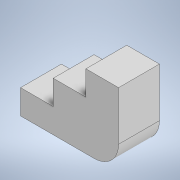
# Autodesk Inventor part: 1.4
Saved by Autodesk Inventor 2022 (Build 260153000, 153)
## iProperties
Created: 2023-04-17
Part Number: 1.4
Material: Genérico
Document SubType Name: Modeling
Designer: jpjoa
Density: 1 g/cm^3
Appearance: Padrão
Author: jpjoa
Autodesk Inventor part; units mm, degrees
ref_plane "YZ Plane" through (0, 0, 0) normal (1, 0, 0) x (0, 1, 0)
ref_plane "XZ Plane" through (0, 0, 0) normal (0, 1, 0) x (-1, 0, 0)
ref_plane "XY Plane" through (0, 0, 0) normal (0, 0, 1) x (1, 0, 0)
sketch "Esboço1" plane through (0, 0, 0) normal (0, 0, 1) x (1, 0, 0)
  line L0 (0, 0) -> (45, 0)
  line L1 (0, 0) -> (0, 15)
  line L2 (0, 15) -> (20, 15)
  line L3 (20, 15) -> (20, 30)
  line L4 (20, 30) -> (40, 30)
  line L5 (40, 30) -> (40, 45)
  line L6 (40, 45) -> (60, 45)
  line L7 (60, 45) -> (60, 15)
  arc A0 (45, 0) -> (60, 15) centre (45, 15) ccw
  point P0 (60, 0)
  dimension "d0" = 60
  dimension "d1" = 15
  dimension "d2" = 20
  dimension "d3" = 15
  dimension "d4" = 20
  dimension "d5" = 15
  dimension "d6" = 20
  dimension "d7" = 15
  constraints: 16 end point, 5 perpendicular, 2 point on circle, 2 point on line, 2 tangent, 1 centre point, 1 horizontal, 1 vertical
  measures "d0" distance of L0.start point (60, 0)
  measures "d1" distance of L0.start L1.end
  measures "d2" distance of L1.end L2.end
  measures "d3" distance of L2.end L3.end
  measures "d4" distance of L3.end L4.end
  measures "d5" distance of L4.end L5.end
  measures "d6" distance of L5.end L6.end
  measures "d7" radius of A0
extrude "Extrusão1" add sketch "Esboço1" along normal blind 25
